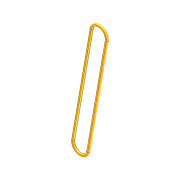
# Autodesk Inventor part: Belt_Vertical_Short
Saved by Autodesk Inventor 2012 (Build 160160000, 160)
## iProperties
Created: 2012-01-13
Part Number: Belt_Vertical_Short
Material: Polypropylene
Document SubType Name: Modeling
Designer: JesseK
Mass: 10.8286 g
Surface Area: 101.048 cm^2
Volume: 12.0451 cm^3
Density: 0.899 g/cm^3
Author: JesseK
Autodesk Inventor part; units mm, degrees
ref_plane "YZ Plane" through (0, 0, 0) normal (1, 0, 0) x (0, 1, 0)
ref_plane "XZ Plane" through (0, 0, 0) normal (0, 1, 0) x (-1, 0, 0)
ref_plane "XY Plane" through (0, 0, 0) normal (0, 0, 1) x (1, 0, 0)
sketch "Sketch1" plane through (0, 0, 0) normal (0, 0, 1) x (1, 0, 0)
  arc A0 (15.6367, -2.7405) -> (-15.6367, 2.7405) centre (0, 0) ccw
  arc A1 (20.3277, -3.5626) -> (-20.3277, 3.5626) centre (0, 0) ccw
  arc A2 (-57.204, -234.4341) -> (-25.9307, -239.9151) centre (-41.5673, -237.1746) ccw
  arc A3 (-61.895, -233.612) -> (-21.2397, -240.7373) centre (-41.5673, -237.1746) ccw
  line L0 (20.3277, -3.5626) -> (-21.2397, -240.7373)
  line L1 (15.6367, -2.7405) -> (-25.9307, -239.9151)
  line L2 (-15.6367, 2.7405) -> (-57.204, -234.4341)
  line L3 (-20.3277, 3.5626) -> (-61.895, -233.612)
  dimension "d0" = 15.875
  dimension "d1" = 4.7625
  constraints: 9 point on circle, 8 end point, 8 tangent, 4 centre point, 3 coincident, 2 parallel
  measures "d0" radius of A0
  measures "d1" radial gap between concentric circles of A0 A1
extrude "Extrusion1" add sketch "Sketch1" along normal blind 4.7625
fillet "Fillet1" radius 2.3813 8 edges at (-45.13, -257.5023, 4.7625) (-41.1113, -115.0247, 4.7625) (3.5626, 20.3277, 4.7625) (-0.456, -122.1499, 4.7625) (3.5626, 20.3277, 0) (-41.1113, -115.0247, 0) (-45.13, -257.5023, 0) (-0.456, -122.1499, 0)
body "Solid1"
